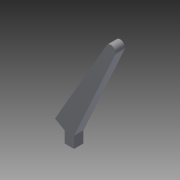
# Autodesk Inventor part: Funneling_v1
Saved by Autodesk Inventor 2013 (Build 170138000, 138)
## iProperties
Created: 2013-01-19
Part Number: Funneling_v1
Material: Generic
Document SubType Name: Modeling
Designer: motoennies
Density: 1 g/cm^3
Author: motoennies
Autodesk Inventor part; units mm, degrees
ref_plane "YZ Plane" through (0, 0, 0) normal (1, 0, 0) x (0, 1, 0)
ref_plane "XZ Plane" through (0, 0, 0) normal (0, 1, 0) x (-1, 0, 0)
ref_plane "XY Plane" through (0, 0, 0) normal (0, 0, 1) x (1, 0, 0)
sketch "Sketch1" plane through (0, 0, 0) normal (0, 0, 1) x (1, 0, 0)
  line L0 (0, 0) -> (0, 7.62)
  line L1 (0, 0) -> (6.35, 0)
  line L2 (0, 7.62) -> (73.3235, 7.62) construction
  line L3 (6.35, 0) -> (6.35, 7.62)
  line L4 (0, 7.62) -> (-6.35, 11.2862)
  line L5 (-6.35, 11.2862) -> (28.1951, 71.12)
  line L6 (28.1951, 71.12) -> (33.6943, 67.945)
  line L7 (33.6943, 67.945) -> (6.35, 7.62)
  arc A0 (33.6943, 67.945) -> (28.1951, 71.12) centre (30.9447, 69.5325) ccw
  dimension "d0" = 7.62
  dimension "d1" = 6.35
  dimension "d8" = 7.62
  dimension "d12" = 6.35
  dimension "d13" = 63.5
  dimension "d14" = 6.35
  dimension "d15" = 120
  constraints: 16 end point, 3 perpendicular, 2 point on circle, 1 centre point, 1 horizontal, 1 midpoint, 1 point on line, 1 vertical
  measures "d0" distance of L0.start L0.end
  measures "d1" distance of L0.start L1.end
  measures "d8" distance of L1.end L3.end
  measures "d12" horizontal distance of L0.start L4.end
  measures "d13" vertical distance of L0.end L5.end
  measures "d14" distance of L5.end L6.end
  measures "d15" angle of L4 L0
extrude "Extrusion2" add sketch "Sketch1" along normal blind 6.35
body "Solid2"
